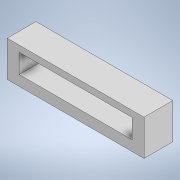
# Autodesk Inventor part: Clip-on
Saved by Autodesk Inventor 2020 (Build 240168000, 168)
## iProperties
Created: 2020-06-06
Part Number: Clip-on
Material: Generic
Document SubType Name: Modeling
Designer: user
Density: 1 g/cm^3
Appearance: Default
PartHeight: 2.500 mm
ClipWidth: 2.900 mm
ClipHeight: 2.500 mm
Author: user
Autodesk Inventor part; units mm, degrees
ref_plane "YZ Plane" through (0, 0, 0) normal (1, 0, 0) x (0, 1, 0)
ref_plane "XZ Plane" through (0, 0, 0) normal (0, 1, 0) x (-1, 0, 0)
ref_plane "XY Plane" through (0, 0, 0) normal (0, 0, 1) x (1, 0, 0)
sketch "Sketch1" plane through (0, 0, 0) normal (0, 1, 0) x (-1, 0, 0)
  line L0 (-19.3909, 30.3636) -> (13.9091, 30.3636)
  line L1 (13.9091, 30.3636) -> (13.9091, 37.3636)
  line L2 (13.9091, 37.3636) -> (-19.3909, 37.3636)
  line L3 (-19.3909, 37.3636) -> (-19.3909, 30.3636)
  point P0 (0, 0)
  dimension "d0" = 33.3
  dimension "d1" = 7
  constraints: 8 end point, 2 parallel, 1 horizontal, 1 perpendicular
  measures "d0" distance of L1.end L2.end
  measures "d1" distance of L0.end L1.end
extrude "MainBody" add sketch "Sketch1" along normal blind 2.5
sketch "Sketch2" plane through (0, 2.5, 0) normal (0, 1, 0) x (1, 0, 0)
  line L0 (-13.9091, -30.3636) -> (-13.9091, -37.3636) projected
  line L1 (-13.9091, -30.3636) -> (-11.0091, -30.3636)
  line L2 (-11.0091, -30.3636) -> (-11.0091, -37.3636)
  line L3 (-11.0091, -37.3636) -> (-13.9091, -37.3636)
  line L4 (-13.9091, -37.3636) -> (-13.9091, -30.3636)
  line L5 (-13.9091, -37.3636) -> (19.3909, -37.3636) projected
  line L6 (19.3909, -37.3636) -> (19.3909, -30.3636) projected
  line L7 (16.4909, -37.3636) -> (19.3909, -37.3636)
  line L8 (19.3909, -37.3636) -> (19.3909, -30.3636)
  line L9 (19.3909, -30.3636) -> (16.4909, -30.3636)
  line L10 (16.4909, -30.3636) -> (16.4909, -37.3636)
  line L11 (19.3909, -30.3636) -> (-13.9091, -30.3636) projected
  point P0 (0, 0)
  point P1 (-13.9091, -37.3636)
  dimension "ClipWidth" = 2.9
  dimension "d5" = 7
  dimension "d14" = 7
  dimension "d15" = 2.9
  dimension "d16" = 0
  dimension "d34" = 27.5
  constraints: 16 end point, 4 parallel, 2 horizontal, 2 perpendicular, 2 point on line
  measures "ClipWidth" distance of L2.end L3.end
  measures "d5" distance of L2.end L1.end
  measures "d14" distance of L9.end L7.start
  measures "d15" distance of L8.end L9.end
  measures "d16" distance from line of L5 L7.start
  measures "d34" distance between parallel lines of L10 L2
extrude "ClipHeight" add sketch "Sketch2" along normal blind 6.2 contours L1 L2 L3 L0 | L9 L6 L5 L10
sketch "Sketch4" plane through (-11.0091, 2.5, 37.3636) normal (1, 0, 0) x (0, 0, -1)
  line L0 (7, 0) -> (7, 6.2) projected
  line L1 (0, 0) -> (0, 6.2) projected
  line L2 (7, 6.2) -> (0, 6.2)
  line L3 (0, 6.2) -> (0, 4.7)
  line L4 (0, 4.7) -> (7, 4.7)
  line L5 (7, 4.7) -> (7, 6.2)
  line L6 (7, 6.2) -> (0, 6.2) projected
  point P0 (37.3636, -2.5)
  dimension "d9" = 1.5
  constraints: 8 end point, 2 parallel, 1 horizontal, 1 perpendicular, 1 point on line
  measures "d9" distance of L3.end L1.end
extrude "Clip1_Out" add sketch "Sketch4" along normal blind 13.85
sketch "Sketch7" plane through (16.4909, 2.5, 30.3636) normal (-1, 0, 0) x (0, 0, 1)
  line L0 (0, 0) -> (0, 6.2) projected
  line L1 (7, 0) -> (7, 6.2) projected
  line L2 (0, 4.7) -> (7, 4.7)
  line L3 (7, 4.7) -> (7, 6.2)
  line L4 (7, 6.2) -> (0, 6.2)
  line L5 (0, 6.2) -> (0, 4.7)
  point P0 (-30.3636, -2.5)
  dimension "d22" = 1.5
  dimension "d23" = 7
  constraints: 8 end point, 2 parallel, 1 horizontal, 1 perpendicular, 1 point on line
  measures "d22" distance of L1.end L2.end
  measures "d23" distance of L1.end L0.end
extrude "Clip2_Out" add sketch "Sketch7" along normal blind 13.65
equation "\"d14\" = d5"
equation "\"d15\" = ClipWidth"
body "Solid1"
